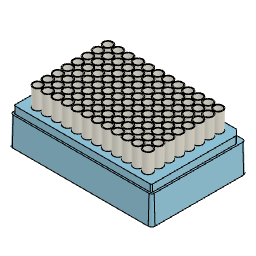
plate dispenser 96 well v6 (Autodesk Fusion 360 archive; units mm, degrees)
design "USA Scientific 1.1 mL strip tubes"
Autodesk Fusion 360 part; units mm, degrees
sketch "Sketch1" plane through (0, 0, 0) normal (0, 0, 1) x (1, 0, 0) in component "Rack MTS-06-C"
  line L0 (61.008, -42.8244) -> (-61.008, -42.8244)
  line L1 (-64.008, -39.8244) -> (-64.008, 39.8244)
  line L2 (-61.008, 42.8244) -> (61.008, 42.8244)
  line L3 (64.008, 39.8244) -> (64.008, -39.8244)
  line L4 (64.008, -42.8244) -> (-64.008, 42.8244) construction
  line L5 (-64.008, -42.8244) -> (64.008, 42.8244) construction
  arc A0 (-61.008, 42.8244) -> (-64.008, 39.8244) centre (-61.008, 39.8244) ccw
  arc A1 (64.008, 39.8244) -> (61.008, 42.8244) centre (61.008, 39.8244) ccw
  arc A2 (61.008, -42.8244) -> (64.008, -39.8244) centre (61.008, -39.8244) ccw
  arc A3 (-64.008, -39.8244) -> (-61.008, -42.8244) centre (-61.008, -39.8244) ccw
  line L6 (60.722, -40.6908) -> (-60.722, -40.6908)
  line L7 (-61.722, -39.6908) -> (-61.722, 39.6908)
  line L8 (-60.722, 40.6908) -> (56.2278, 40.6908)
  line L9 (61.722, 35.1966) -> (61.722, -39.6908)
  line L10 (61.722, -40.6908) -> (-61.722, 40.6908) construction
  line L11 (-61.722, -40.6908) -> (61.722, 40.6908) construction
  arc A4 (-60.722, 40.6908) -> (-61.722, 39.6908) centre (-60.722, 39.6908) ccw
  arc A5 (61.722, 39.6908) -> (60.722, 40.6908) centre (60.722, 39.6908) ccw
  arc A6 (60.722, -40.6908) -> (61.722, -39.6908) centre (60.722, -39.6908) ccw
  arc A7 (-61.722, -39.6908) -> (-60.722, -40.6908) centre (-60.722, -39.6908) ccw
  line L12 (56.9349, 40.3979) -> (61.4291, 35.9037)
  arc A8 (56.9349, 40.3979) -> (56.2278, 40.6908) centre (56.2278, 39.6908) ccw
  arc A9 (61.722, 35.1966) -> (61.4291, 35.9037) centre (60.722, 35.1966) ccw
  point P0 (56.642, 40.6908)
  dimension "d12" = 128.016
  dimension "d13" = 85.6488
  dimension "d14" = 3
  dimension "d15" = 3
  dimension "d16" = 3
  dimension "d17" = 123.444
  dimension "d18" = 81.3816
  dimension "d19" = 1
  dimension "d27" = 5.08
  dimension "d28" = 45
  dimension "d29" = 1
  constraint horizontal L0
  constraint perpendicular L0 L1
  constraint parallel L0 L2
  constraint parallel L1 L3
  constraint coincident L4 origin
  constraint coincident L5 origin
  constraint coincident L4.end L1
  constraint coincident L4.end L2
  constraint tangent L1 A0
  constraint tangent L2 A0
  constraint coincident L5.end L3
  constraint coincident L5.end L2
  constraint tangent L3 A1
  constraint tangent L2 A1
  constraint coincident L4.start L3
  constraint coincident L4.start L0
  constraint tangent L3 A2
  constraint tangent L0 A2
  constraint equal A1 A2
  constraint coincident L5.start L1
  constraint coincident L5.start L0
  constraint tangent L1 A3
  constraint tangent L0 A3
  constraint horizontal L6
  constraint perpendicular L6 L7
  constraint parallel L6 L8
  constraint parallel L7 L9
  constraint coincident L10 origin
  constraint coincident L11 origin
  constraint coincident L10.end L7
  constraint coincident L10.end L8
  constraint tangent L7 A4
  constraint tangent L8 A4
  constraint coincident L11.end L8
  constraint coincident L11.end L9
  constraint tangent L8 A5
  constraint tangent L9 A5
  constraint equal A4 A5
  constraint coincident L10.start L9
  constraint coincident L10.start L6
  constraint tangent L9 A6
  constraint tangent L6 A6
  constraint equal A4 A6
  constraint coincident L11.start L7
  constraint coincident L11.start L6
  constraint tangent L7 A7
  constraint tangent L6 A7
  constraint equal A4 A7
  constraint coincident L8 P0
  constraint coincident P0 L12
  constraint coincident L8 A5.end
  constraint tangent L12 A8
  constraint tangent L8 A8
  constraint coincident L9 A5.start
  constraint tangent L9 A9
  constraint tangent L12 A9
  constraint equal A8 A9
  measures "d12" distance of L4.end L5.end
  measures "d13" distance of L5.start L4.end
  measures "d14" radius of A0
  measures "d15" radius of A1
  measures "d16" radius of A3
  measures "d17" distance of L10.end L11.end
  measures "d18" distance of L11.start L10.end
  measures "d19" radius of A4
  measures "d27" distance of L9 P0
  measures "d28" angle of L8 L12
  measures "d29" radius of A8
extrude "Extrude1" add sketch "Sketch1" along normal blind 31.623 contours L6 L7 L8 L9 A4 A6 A7 L12 A8 A9 makes body 1 in component "Rack MTS-06-C"
extrude "Extrude2" add sketch "Sketch1" along normal blind 25.273 draft -1.5 contours L0 L1 L2 L3 A0 A1 A2 A3 | L6 L7 L8 L9 A4 A6 A7 L12 A8 A9 bodies 1 in component "Rack MTS-06-C"
sketch "Sketch2" plane through (0, 0, 31.623) normal (0, 0, 1) x (-1, 0, 0) in component "Rack MTS-06-C"
  circle A0 centre (49.4995, -31.5011) radius 4.0513
  circle A1 centre (40.4996, -31.5011) radius 4.0513
  circle A2 centre (31.4997, -31.5011) radius 4.0513
  circle A3 centre (22.4998, -31.5011) radius 4.0513
  circle A4 centre (13.4999, -31.5011) radius 4.0513
  circle A5 centre (4.5, -31.5011) radius 4.0513
  circle A6 centre (-4.5, -31.5011) radius 4.0513
  circle A7 centre (-13.4999, -31.5011) radius 4.0513
  circle A8 centre (-22.4998, -31.5011) radius 4.0513
  circle A9 centre (-31.4997, -31.5011) radius 4.0513
  circle A10 centre (-40.4996, -31.5011) radius 4.0513
  circle A11 centre (-49.4995, -31.5011) radius 4.0513
  circle A12 centre (49.4995, -22.5008) radius 4.0513
  circle A13 centre (40.4996, -22.5008) radius 4.0513
  circle A14 centre (31.4997, -22.5008) radius 4.0513
  circle A15 centre (22.4998, -22.5008) radius 4.0513
  circle A16 centre (13.4999, -22.5008) radius 4.0513
  circle A17 centre (4.5, -22.5008) radius 4.0513
  circle A18 centre (-4.5, -22.5008) radius 4.0513
  circle A19 centre (-13.4999, -22.5008) radius 4.0513
  circle A20 centre (-22.4998, -22.5008) radius 4.0513
  circle A21 centre (-31.4997, -22.5008) radius 4.0513
  circle A22 centre (-40.4996, -22.5008) radius 4.0513
  circle A23 centre (-49.4995, -22.5008) radius 4.0513
  circle A24 centre (49.4995, -13.5005) radius 4.0513
  circle A25 centre (40.4996, -13.5005) radius 4.0513
  circle A26 centre (31.4997, -13.5005) radius 4.0513
  circle A27 centre (22.4998, -13.5005) radius 4.0513
  circle A28 centre (13.4999, -13.5005) radius 4.0513
  circle A29 centre (4.5, -13.5005) radius 4.0513
  circle A30 centre (-4.5, -13.5005) radius 4.0513
  circle A31 centre (-13.4999, -13.5005) radius 4.0513
  circle A32 centre (-22.4998, -13.5005) radius 4.0513
  circle A33 centre (-31.4997, -13.5005) radius 4.0513
  circle A34 centre (-40.4996, -13.5005) radius 4.0513
  circle A35 centre (-49.4995, -13.5005) radius 4.0513
  circle A36 centre (49.4995, -4.5002) radius 4.0513
  circle A37 centre (40.4996, -4.5002) radius 4.0513
  circle A38 centre (31.4997, -4.5002) radius 4.0513
  circle A39 centre (22.4998, -4.5002) radius 4.0513
  circle A40 centre (13.4999, -4.5002) radius 4.0513
  circle A41 centre (4.5, -4.5002) radius 4.0513
  circle A42 centre (-4.5, -4.5002) radius 4.0513
  circle A43 centre (-13.4999, -4.5002) radius 4.0513
  circle A44 centre (-22.4998, -4.5002) radius 4.0513
  circle A45 centre (-31.4997, -4.5002) radius 4.0513
  circle A46 centre (-40.4996, -4.5002) radius 4.0513
  circle A47 centre (-49.4995, -4.5002) radius 4.0513
  circle A48 centre (49.4995, 4.5002) radius 4.0513
  circle A49 centre (40.4996, 4.5002) radius 4.0513
  circle A50 centre (31.4997, 4.5002) radius 4.0513
  circle A51 centre (22.4998, 4.5002) radius 4.0513
  circle A52 centre (13.4999, 4.5002) radius 4.0513
  circle A53 centre (4.5, 4.5002) radius 4.0513
  circle A54 centre (-4.5, 4.5002) radius 4.0513
  circle A55 centre (-13.4999, 4.5002) radius 4.0513
  circle A56 centre (-22.4998, 4.5002) radius 4.0513
  circle A57 centre (-31.4997, 4.5002) radius 4.0513
  circle A58 centre (-40.4996, 4.5002) radius 4.0513
  circle A59 centre (-49.4995, 4.5002) radius 4.0513
  circle A60 centre (49.4995, 13.5005) radius 4.0513
  circle A61 centre (40.4996, 13.5005) radius 4.0513
  circle A62 centre (31.4997, 13.5005) radius 4.0513
  circle A63 centre (22.4998, 13.5005) radius 4.0513
  circle A64 centre (13.4999, 13.5005) radius 4.0513
  circle A65 centre (4.5, 13.5005) radius 4.0513
  circle A66 centre (-4.5, 13.5005) radius 4.0513
  circle A67 centre (-13.4999, 13.5005) radius 4.0513
  circle A68 centre (-22.4998, 13.5005) radius 4.0513
  circle A69 centre (-31.4997, 13.5005) radius 4.0513
  circle A70 centre (-40.4996, 13.5005) radius 4.0513
  circle A71 centre (-49.4995, 13.5005) radius 4.0513
  circle A72 centre (49.4995, 22.5008) radius 4.0513
  circle A73 centre (40.4996, 22.5008) radius 4.0513
  circle A74 centre (31.4997, 22.5008) radius 4.0513
  circle A75 centre (22.4998, 22.5008) radius 4.0513
  circle A76 centre (13.4999, 22.5008) radius 4.0513
  circle A77 centre (4.5, 22.5008) radius 4.0513
  circle A78 centre (-4.5, 22.5008) radius 4.0513
  circle A79 centre (-13.4999, 22.5008) radius 4.0513
  circle A80 centre (-22.4998, 22.5008) radius 4.0513
  circle A81 centre (-31.4997, 22.5008) radius 4.0513
  circle A82 centre (-40.4996, 22.5008) radius 4.0513
  circle A83 centre (-49.4995, 22.5008) radius 4.0513
  circle A84 centre (49.4995, 31.5011) radius 4.0513
  circle A85 centre (40.4996, 31.5011) radius 4.0513
  circle A86 centre (31.4997, 31.5011) radius 4.0513
  circle A87 centre (22.4998, 31.5011) radius 4.0513
  circle A88 centre (13.4999, 31.5011) radius 4.0513
  circle A89 centre (4.5, 31.5011) radius 4.0513
  circle A90 centre (-4.5, 31.5011) radius 4.0513
  circle A91 centre (-13.4999, 31.5011) radius 4.0513
  circle A92 centre (-22.4998, 31.5011) radius 4.0513
  circle A93 centre (-31.4997, 31.5011) radius 4.0513
  circle A94 centre (-40.4996, 31.5011) radius 4.0513
  circle A95 centre (-49.4995, 31.5011) radius 4.0513
  dimension "d30" = 8.1026
  dimension "d31" = 49.4995
  dimension "d32" = 31.5011
  dimension "d35" = -98.999
  dimension "d36" = 63.0022
  measures "d30" diameter of A0
  measures "d31" horizontal distance of origin A0.centre
  measures "d32" vertical distance of origin A0.centre
shell "Shell1" thickness 1 removed faces 0 bodies 1 in component "Rack MTS-06-C"
extrude "Extrude3" cut sketch "Sketch2" against normal blind 30.623 bodies 1 in component "Rack MTS-06-C"
sketch "Sketch1 (2)" plane through (0, 0, 0) normal (0, 1, 0) x (1, 0, 0) in component "Tube MTS-11-C-R"
  line L0 (0, 0) -> (0, 45.466)
  line L1 (0, 0) -> (4.2672, 0)
  line L2 (4.2672, 0) -> (3.3909, 43.4663)
  line L3 (0.3397, 46.4566) -> (0, 46.4566)
  arc A0 (3.3909, 43.4663) -> (0.3397, 46.4566) centre (0.3397, 43.4048) ccw
  line L4 (0, 46.4566) -> (0, 45.466)
  line L5 (4.2672, 0) -> (4.1275, 17.3482)
  line L6 (4.1275, 17.3482) -> (3.9175, 17.3482)
  line L7 (3.5052, 0) -> (2.6193, 43.9445)
  line L8 (1.0668, 45.466) -> (0, 45.466)
  arc A1 (2.6193, 43.9445) -> (1.0668, 45.466) centre (1.0668, 43.9132) ccw
  dimension "d44" = 45.466
  dimension "d45" = 4.2672
  dimension "d46" = 46.4566
  dimension "d48" = 3.0518
  dimension "d50" = 3.3909
  dimension "d52" = 4.1275
  dimension "d53" = 17.3482
  dimension "d55" = 45.466
  dimension "d56" = 3.5052
  dimension "d57" = 1.5528
  constraint coincident L0.start L1.start
  constraint vertical L0
  constraint perpendicular L0 L1
  constraint horizontal L3
  constraint tangent L3 A0
  constraint tangent L2 A0
  constraint vertical L0.end L3.end
  constraint parallel L1 L6
  constraint coincident L1 L7.start
  constraint parallel L2 L7
  constraint coincident L0 L4.end
  constraint perpendicular L0 L8
  constraint tangent L7 A1
  constraint tangent L8 A1
  constraint coincident L2 L6.end
  measures "d44" distance of L0.start L0.end
  measures "d45" distance of L0.start L1.end
  measures "d46" distance of L0.start L3.end
  measures "d48" radius of A0
  measures "d50" distance of L0 L2.end
  measures "d52" distance of L0 L5.end
  measures "d53" distance of L1 L5.end
  measures "d55" distance of L1 L8
  measures "d56" distance of L0.start L7.start
  measures "d57" radius of A1
revolve "Revolve1" add sketch "Sketch1 (2)" angle 360 about axis through (0, 0, 0) along (0, 0, -1) separate body contours L1 L2 L3 A0 L4 L7 L8 A1 | L2 L5 L6 makes body 2 in component "Tube MTS-11-C-R"
pattern_linear "礁8" [suppressed] in component "Tube strip"
pattern_linear "爁8" [suppressed]
component "Rack MTS-06-C" placed x (1, 0, 0) y (0, 1, 0) z (0, 0, 1) at (0, 0, 0)
component "Tube strip" placed x (1, 0, 0) y (0, 1, 0) z (0, 0, 1) at (0, 0, 0)
component "Tube strip" placed x (1, 0, 0) y (0, 1, 0) z (0, 0, 1) at (9, 0, 0)
component "Tube strip" placed x (1, 0, 0) y (0, 1, 0) z (0, 0, 1) at (18, 0, 0)
component "Tube strip" placed x (1, 0, 0) y (0, 1, 0) z (0, 0, 1) at (27, 0, 0)
component "Tube strip" placed x (1, 0, 0) y (0, 1, 0) z (0, 0, 1) at (36, 0, 0)
component "Tube strip" placed x (1, 0, 0) y (0, 1, 0) z (0, 0, 1) at (45, 0, 0)
component "Tube strip" placed x (1, 0, 0) y (0, 1, 0) z (0, 0, 1) at (54, 0, 0)
component "Tube strip" placed x (1, 0, 0) y (0, 1, 0) z (0, 0, 1) at (63, 0, 0)
component "Tube strip" placed x (1, 0, 0) y (0, 1, 0) z (0, 0, 1) at (72, 0, 0)
component "Tube strip" placed x (1, 0, 0) y (0, 1, 0) z (0, 0, 1) at (81, 0, 0)
component "Tube strip" placed x (1, 0, 0) y (0, 1, 0) z (0, 0, 1) at (90, 0, 0)
component "Tube strip" placed x (1, 0, 0) y (0, 1, 0) z (0, 0, 1) at (99, 0, 0)
component "Tube MTS-11-C-R" placed x (1, 0, 0) y (0, 1, 0) z (0, 0, 1) at (-49.4995, 31.5011, 48.9712) in component "Tube strip"
component "Tube MTS-11-C-R" placed x (1, 0, 0) y (0, 1, 0) z (0, 0, 1) at (-49.4995, 22.5008, 48.9712) in component "Tube strip"
component "Tube MTS-11-C-R" placed x (1, 0, 0) y (0, 1, 0) z (0, 0, 1) at (-49.4995, 13.5005, 48.9712) in component "Tube strip"
component "Tube MTS-11-C-R" placed x (1, 0, 0) y (0, 1, 0) z (0, 0, 1) at (-49.4995, 4.5002, 48.9712) in component "Tube strip"
component "Tube MTS-11-C-R" placed x (1, 0, 0) y (0, 1, 0) z (0, 0, 1) at (-49.4995, -4.5002, 48.9712) in component "Tube strip"
component "Tube MTS-11-C-R" placed x (1, 0, 0) y (0, 1, 0) z (0, 0, 1) at (-49.4995, -13.5005, 48.9712) in component "Tube strip"
component "Tube MTS-11-C-R" placed x (1, 0, 0) y (0, 1, 0) z (0, 0, 1) at (-49.4995, -22.5008, 48.9712) in component "Tube strip"
component "Tube MTS-11-C-R" placed x (1, 0, 0) y (0, 1, 0) z (0, 0, 1) at (-49.4995, -31.5011, 48.9712) in component "Tube strip"
equation "base_length = 5.0400 in"
equation "base_lip_height = 0.9950 in"
equation "base_height = 1.245 in"
equation "base_top_width = 3.2040 in"
equation "base_width = 3.3720 in"
equation "base_top_length = 4.8600 in"
equation "base_well_A1_X_offset_center = 1.9488 in"
equation "base_well_A1_Y_offset_center = 1.2402 in"
equation "base_well_dia = 0.3190 in"
equation "base_fillet_rad = 3 mm"
equation "base_top_fillet_rad = 1 mm"
equation "d12 = base_length"
equation "d13 = base_width"
equation "d14 = base_fillet_rad"
equation "d15 = base_fillet_rad"
equation "d16 = base_fillet_rad"
equation "d17 = base_top_length"
equation "d18 = base_top_width"
equation "d19 = base_top_fillet_rad"
equation "d20 = base_height"
equation "base_flange_draft_angle = -1.5 deg"
equation "d23 = base_lip_height"
equation "d24 = base_flange_draft_angle"
equation "base_corner_cut_length = 0.2 in"
equation "d27 = base_corner_cut_length"
equation "d29 = base_top_fillet_rad"
equation "d30 = base_well_dia"
equation "d31 = base_well_A1_X_offset_center"
equation "d32 = base_well_A1_Y_offset_center"
equation "d35 = -( 2 * base_well_A1_X_offset_center )"
equation "d36 = 2 * ( base_well_A1_Y_offset_center )"
equation "d37 = -( base_height - 1 mm )"
equation "tube_top_ID = 0.276 in"
equation "tube_top_OD = 0.336 in"
equation "tube_outside_height = 1.829 in"
equation "tube_inside_height = 1.790 in"
equation "tube_lip_height = 0.683 in"
equation "d44 = tube_inside_height"
equation "d45 = tube_top_OD / 2"
equation "d46 = tube_outside_height"
equation "tube_bottom_od = 0.267 in"
equation "d48 = ( tube_bottom_od * 0.9 ) / 2"
equation "d50 = tube_bottom_od / 2"
equation "tube_lip_OD = 0.325 in"
equation "d52 = tube_lip_OD / 2"
equation "d53 = tube_lip_height"
equation "d55 = tube_inside_height"
equation "d56 = tube_top_ID / 2"
equation "d73 = 2 * base_well_A1_Y_offset_center"
